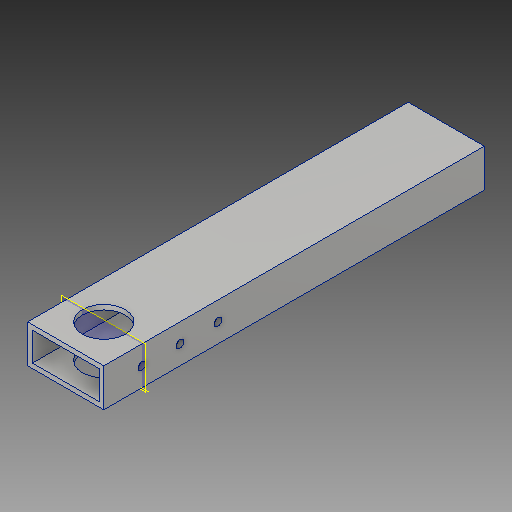
# Autodesk Inventor part: 15102898-16-A-0201
Saved by Autodesk Inventor 2017 (Build 210142000, 142)
## iProperties
Created: 2016-09-26
Part Number: 15102898-16-A-0201
Material: Aluminum 6061
Document SubType Name: Modeling
Designer: gus
Density: 2.7 g/cm^3
Appearance: Aluminum - Flat
Mass: 292.114 g
Surface Area: 699.174 cm^2
Volume: 108.191 cm^3
Author: gus
Autodesk Inventor part; units mm, degrees
ref_plane "YZ Plane" through (0, 0, 0) normal (1, 0, 0) x (0, 1, 0)
ref_plane "XZ Plane" through (0, 0, 0) normal (0, 1, 0) x (-1, 0, 0)
ref_plane "XY Plane" through (0, 0, 0) normal (0, 0, 1) x (1, 0, 0)
sketch "Sketch1" plane through (0, 0, 0) normal (0, 0, 1) x (1, 0, 0)
  line L0 (0, 0) -> (50.8, 0)
  line L1 (50.8, 0) -> (50.8, 25.4)
  line L2 (50.8, 25.4) -> (0, 25.4)
  line L3 (0, 25.4) -> (0, 0)
  line L4 (3.175, 22.225) -> (47.625, 22.225)
  line L5 (47.625, 22.225) -> (47.625, 3.175)
  line L6 (47.625, 3.175) -> (3.175, 3.175)
  line L7 (3.175, 3.175) -> (3.175, 22.225)
  dimension "d0" = 50.8
  dimension "d1" = 25.4
  dimension "d2" = 3.175
  constraints: 16 end point, 4 parallel, 2 perpendicular, 1 horizontal, 3 other
  measures "d0" distance of L2.end L1.end
  measures "d1" distance of L1.end L0.end
  measures "d2" distance between parallel lines of L2 L4
extrude "Extrusion1" add sketch "Sketch1" along normal blind 254
sketch "Sketch2" plane through (0, 0, 0) normal (0, -1, 0) x (1, 0, 0)
  circle A0 centre (25.4, 228.6) radius 4.7625
  line L0 (47.625, 254) -> (3.175, 254) projected
  line L1 (0, 0) -> (0, 254) projected
  dimension "d5" = 9.525
  dimension "d6" = 25.4
  dimension "d7" = 25.4
  constraints: 1 centre point
  measures "d5" diameter of A0
  measures "d6" distance from line of L0 A0.centre
  measures "d7" distance from line of L1 A0.centre
extrude "Extrusion2" cut sketch "Sketch2" against normal blind 25.4
sketch "Sketch3" plane through (0, 25.4, 0) normal (0, 1, 0) x (1, 0, 0)
  circle A0 centre (25.4, -228.6) radius 4.7625 projected
  circle A1 centre (25.4, -228.6) radius 14.2875
  point P0 (0, 0)
  dimension "d10" = 28.575
  constraints: 1 centre point, 1 coincident
  measures "d10" diameter of A1
extrude "Extrusion3" cut sketch "Sketch3" against normal blind 25.4
ref_plane "Work Plane1" through (25.4, 0, 228.6) normal (0, 0, -1) x (1, 0, 0)
sketch "Sketch5" plane through (50.8, 0, 0) normal (1, 0, 0) x (0, 0, -1)
  line L0 (-254, 0) -> (-254, 25.4) projected
  line L1 (0, 0) -> (-254, 0) projected
  line L2 (0, 25.4) -> (-254, 25.4) projected
  point P0 (-228.6, 12.7)
  point P1 (-203.2, 12.7)
  point P2 (-177.8, 12.7)
  dimension "d21" = 25.4
  dimension "d22" = 12.7
  dimension "d23" = 25.4
  dimension "d24" = 25.4
  dimension "d25" = 12.7
  dimension "d26" = 12.7
  measures "d21" distance from line of L0 point (-228.6, 12.7)
  measures "d22" distance from line of L1 point (-228.6, 12.7)
  measures "d23" distance of point (-203.2, 12.7) point (-228.6, 12.7)
  measures "d24" distance of point (-177.8, 12.7) point (-203.2, 12.7)
  measures "d25" distance from line of L2 point (-203.2, 12.7)
  measures "d26" distance from line of L2 point (-177.8, 12.7)
hole "Hole1" at (50.8, 12.7, 228.6) at (50.8, 12.7, 203.2) at (50.8, 12.7, 177.8) direction (-1, 0, 0) diameter 5.1594 end through all
thread "Thread1" size "12-24 UNC" class "2B" standard "ANSI Unified Screw Threads" full length
thread "Thread2" size "12-24 UNC" class "2B" standard "ANSI Unified Screw Threads" full length
thread "Thread3" size "12-24 UNC" class "2B" standard "ANSI Unified Screw Threads" full length
body "Solid1"
